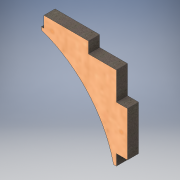
# Autodesk Inventor part: protector
Saved by Autodesk Inventor 2019 (Build 230136000, 136)
## iProperties
Created: 2020-12-06
Part Number: protector
Material: Дерево (береза)
Document SubType Name: Modeling
Designer: Professional
Density: 0.55 g/cm^3
Appearance: Береза — натуральный — полированный
Author: Professional
Autodesk Inventor part; units mm, degrees
ref_plane "YZ Plane" through (0, 0, 0) normal (1, 0, 0) x (0, 1, 0)
ref_plane "XZ Plane" through (0, 0, 0) normal (0, 1, 0) x (-1, 0, 0)
ref_plane "XY Plane" through (0, 0, 0) normal (0, 0, 1) x (1, 0, 0)
sketch "Эскиз1" plane through (0, 0, 0) normal (0, 0, 1) x (1, 0, 0)
  line L0 (0, 0) -> (0, -10)
  line L1 (0, -10) -> (4, -10)
  line L2 (4, -10) -> (4, -26)
  line L3 (4, -26) -> (0, -26)
  line L4 (0, -26) -> (0, -29.9118)
  line L5 (0, -29.9118) -> (-1, -29.9118)
  arc A0 (-1, -29.9118) -> (-26.9172, -1) centre (-40, -38.8) ccw
  line L6 (-26.9172, -1) -> (-26.9172, 0)
  line L7 (-26.9172, 0) -> (-26, 0)
  line L8 (-26, 0) -> (-26, 4)
  line L9 (-26, 4) -> (-10, 4)
  line L10 (-10, 4) -> (-10, 0)
  line L11 (-10, 0) -> (0, 0)
  dimension "d0" = 40
  dimension "d1" = 1
  dimension "d3" = 38.8
  dimension "d4" = 4
  dimension "d5" = 40
  dimension "d6" = 16
  dimension "d7" = 10
  dimension "d8" = 16
  dimension "d9" = 10
  constraints: 24 end point, 10 perpendicular, 3 point on line, 2 point on circle, 2 vertical, 1 centre point, 1 horizontal
  measures "d0" radius of A0
  measures "d1" distance of L4.end L5.end
  measures "d3" distance from line of L7 A0.centre
  measures "d4" distance of L9.end L10.end
  measures "d5" distance from line of A0.centre L4
  measures "d6" distance of L1.end L2.end
  measures "d7" distance between parallel lines of L11 L1
  measures "d8" distance between parallel lines of L10 L8
  measures "d9" distance from line of L0.start L10
extrude "Выдавливание1" add sketch "Эскиз1" along normal blind 4
